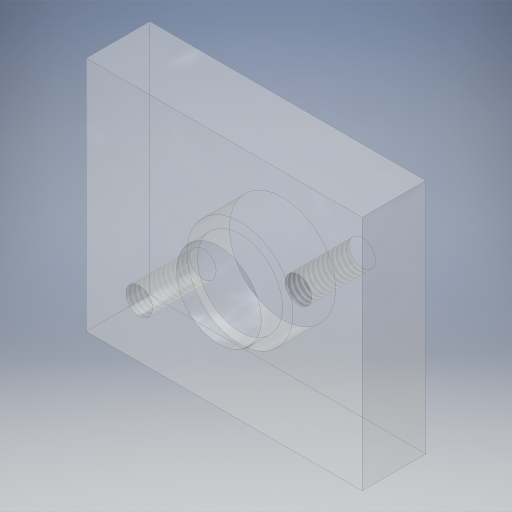
# Autodesk Inventor part: BT804_goteln20_22
Saved by Autodesk Inventor 2023 (Build 270158000, 158)
## iProperties
Company: HTBLA Kaindorf
RuleStatus: InUse
Created: 2023-01-12
Part Number: BT804_goteln20_22
Project: Zeichenmaschine_neu
Material: Acryl
Description: getriebe_lagerung
Document SubType Name: Modeling
Designer: goteln20
Density: 1.188 g/cm^3
Appearance: Transparent - farblos
Mass: 3.57018 g
Surface Area: 18.8921 cm^2
Volume: 3.0052 cm^3
AfterDocNew0: iProperties-Editor_aufrufen
Author: eligo
Keywords: 22
Autodesk Inventor part; units mm, degrees
ref_plane "YZ Plane" through (0, 0, 0) normal (1, 0, 0) x (0, 1, 0)
ref_plane "XZ Plane" through (0, 0, 0) normal (0, 1, 0) x (-1, 0, 0)
ref_plane "XY Plane" through (0, 0, 0) normal (0, 0, 1) x (1, 0, 0)
derived "BT803_goteln20_22_Zeichenmaschine_neu_getriebe.ipt"
sketch "Skizze4" plane through (0, -32, 22.3) normal (1, 0, 0) x (0, 0, -1)
  line L0 (21.4184, 32) -> (0, 32)
  line L1 (0, 0) -> (0, 32)
  line L2 (22.3, 5) -> (22.3, 27)
  line L3 (21.4184, 0) -> (0, 0)
  point P0 (22.3, 32)
  point P1 (8.9, 26)
  point P2 (17.3, 11)
  point P3 (13.1, 18.5)
sketch "Skizze5" plane through (0, 0, 0) normal (1, 0, 0) x (0, 1, 0)
  line L0 (-26, 0) -> (-26, 22.3)
  line L1 (-32, 22.3) -> (0, 22.3) projected
  line L2 (-27, 0) -> (-5, 0) projected
  line L3 (-26, 0) -> (0, 0)
  line L4 (-32, 0.8816) -> (-32, 22.3) projected
  line L5 (0, 0) -> (0, 22.3)
  line L6 (0, 0.1273) -> (0, 0)
  point P0 (-6, 13.4)
  point P1 (-13.5, 9.2)
  point P2 (-21, 5)
  dimension "d5" = 6
  constraints: 8 end point, 2 point on line, 2 vertical, 1 collinear, 1 horizontal
  measures "d5" distance between parallel lines of L4 L0
extrude "Extrusion3" add sketch "Skizze5" along normal blind 6
hole "Bohrung1" at (0, -6, 13.4) at (0, -21, 5) direction (1, 0, 0) diameter 2.5 depth 8
thread "Gewinde1" size "M2.5x0.45" class "6H" standard "ISO Metric profile" length 8
thread "Gewinde2" size "M2.5x0.45" class "6H" standard "ISO Metric profile" length 8
hole "Bohrung2" at (0, -13.5, 9.2) direction (1, 0, 0) diameter 8 depth 8 counterbore diameter 10 counterbore depth 4
